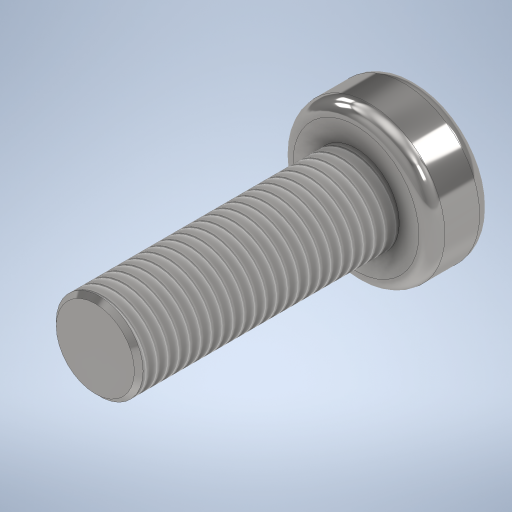
# Autodesk Inventor part: 십자 둥근머리 볼트 6mm
Saved by Autodesk Inventor 2023 (Build 270158000, 158)
## iProperties
Created: 2022-06-06
Part Number: 십자 둥근머리 볼트 6mm
Material: 일반
Document SubType Name: Modeling
Designer: fly01
Density: 1 g/cm^3
Appearance: 기본값
Author: fly01
Autodesk Inventor part; units mm, degrees
ref_plane "YZ Plane" through (0, 0, 0) normal (1, 0, 0) x (0, 1, 0)
ref_plane "XZ Plane" through (0, 0, 0) normal (0, 1, 0) x (-1, 0, 0)
ref_plane "XY Plane" through (0, 0, 0) normal (0, 0, 1) x (1, 0, 0)
sketch "스케치1" plane through (0, 0, 0) normal (0, 0, 1) x (1, 0, 0)
  circle A0 centre (0, 0) radius 1
  circle A1 centre (0, 0) radius 1.75
  dimension "d0" = 2
  dimension "d3" = 3.5
  constraints: 2 centre point, 2 coincident
  measures "d0" diameter of A0
  measures "d3" diameter of A1
extrude "돌출1" add sketch "스케치1" along normal blind 6 contours A0
extrude "돌출2" add sketch "스케치1" against normal blind 1.4 contours A0 | A1
fillet "모깎기1" radius 0.3 2 edges at (-1.75, 0, 0) (-1.75, 0, -1.4)
sketch "스케치2" plane through (0, 0, -1.4) normal (0, 0, -1) x (-1, 0, 0)
  line L0 (-0.25, -1) -> (0.25, -1)
  line L1 (0.25, -1) -> (0.25, 1)
  line L2 (0.25, 1) -> (-0.25, 1)
  line L3 (-0.25, 1) -> (-0.25, -1)
  line L4 (-0.25, -1) -> (0.25, 1) construction
  line L5 (0.25, -1) -> (-0.25, 1) construction
  line L6 (-1, -0.25) -> (1, -0.25)
  line L7 (1, -0.25) -> (1, 0.25)
  line L8 (1, 0.25) -> (-1, 0.25)
  line L9 (-1, 0.25) -> (-1, -0.25)
  line L10 (-1, -0.25) -> (1, 0.25) construction
  line L11 (1, -0.25) -> (-1, 0.25) construction
  point P0 (0, 0)
  point P1 (0.25, 0.25)
  point P2 (-0.25, 0.25)
  point P3 (0.25, -0.25)
  point P4 (-0.25, -0.25)
  dimension "d7" = 0.5
  dimension "d8" = 2
  dimension "d9" = 2
  dimension "d10" = 0.5
  constraints: 24 end point, 4 midpoint, 4 parallel, 2 horizontal, 2 perpendicular
  measures "d7" distance of L2.end L1.end
  measures "d8" distance of L1.end L0.end
  measures "d9" distance of L8.end L7.end
  measures "d10" distance of L7.end L6.end
extrude "돌출3" cut sketch "스케치2" against normal blind 0.7
chamfer "모따기1" distance 0.1 angle 45 1 edges at (-1, 0, 6)
thread "스레드1" size "M2x0.25" class "6g" standard "ANSI Metric M Profile" full length
